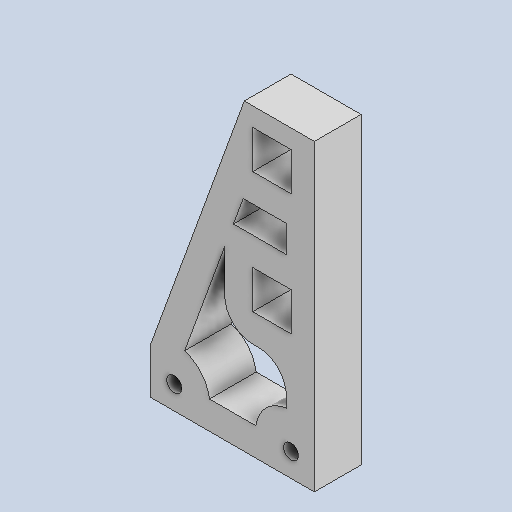
# Autodesk Inventor part: Soporte lateral
Saved by Autodesk Inventor 2024 (Build 280153000, 153)
## iProperties
Created: 2025-03-01
Part Number: Soporte lateral
Material: Genérico
Document SubType Name: Modeling
Designer: sergi
Density: 1 g/cm^3
Appearance: Valor por defecto
Author: sergi
Autodesk Inventor part; units mm, degrees
ref_plane "YZ Plane" through (0, 0, 0) normal (1, 0, 0) x (0, 1, 0)
ref_plane "XZ Plane" through (0, 0, 0) normal (0, 1, 0) x (-1, 0, 0)
ref_plane "XY Plane" through (0, 0, 0) normal (0, 0, 1) x (1, 0, 0)
sketch "Boceto1" plane through (0, 0, 0) normal (0, 0, 1) x (1, 0, 0)
  line L0 (0, 0) -> (105, 0)
  line L1 (105, 0) -> (105, 55)
  line L2 (105, 55) -> (0, 0)
  line L3 (105, 55) -> (90, 55)
  line L4 (90, 55) -> (0, 0)
  line L5 (0, 0) -> (70, 0)
  line L6 (70, 0) -> (90, 55)
  dimension "d0" = 105
  dimension "d1" = 55
  dimension "d4" = 15
  dimension "d10" = 70
  constraints: 14 end point, 2 horizontal, 1 perpendicular, 1 point on line
  measures "d0" distance of L0.start L0.end
  measures "d1" distance of L0.end L1.end
  measures "d4" distance of L1.end L3.end
  measures "d10" distance of L0.start L5.end
extrude "Extrusión1" add sketch "Boceto1" along normal blind 10 contours L6 L2 L1 L0 | L6 L3 L2
sketch "Boceto2" plane through (0, 0, 10) normal (0, 0, 1) x (1, 0, 0)
  line L0 (-10.0369, 16.82) -> (-5.1631, 16.82) projected
  line L1 (-1.5564, 16.82) -> (-5.1631, 16.82) projected
  line L2 (-1.5564, 16.82) -> (105, 16.82)
  line L3 (105, 0) -> (105, 55) projected
  line L4 (105, 55) -> (90, 55) projected
  line L5 (70, 0) -> (105, 0) projected
  line L6 (100, 5) -> (14.5727, 5)
  line L7 (90, 55) -> (70, 0) projected
  line L8 (105, 55) -> (105, 42.8)
  line L9 (105, 55) -> (117.2, 55) construction
  line L10 (70, 0) -> (105, 0) projected
  line L11 (105, 0) -> (105, 16.82)
  line L12 (105, 0) -> (105, 55) projected
  line L13 (105, 16.82) -> (100, 16.82)
  line L14 (100, 16.82) -> (94.1, 16.82)
  line L15 (94.1, 16.82) -> (94.1, 25.02)
  line L16 (94.1, 25.02) -> (100, 25.02)
  line L17 (100, 25.02) -> (100, 16.82)
  line L18 (105, 42.8) -> (100, 42.8)
  line L19 (100, 42.8) -> (91.8, 42.8)
  line L20 (91.8, 42.8) -> (91.8, 51)
  line L21 (91.8, 51) -> (100, 51)
  line L22 (100, 51) -> (100, 42.8)
  line L23 (100, 16.82) -> (91.8, 16.82)
  line L24 (91.8, 16.82) -> (91.8, 25.02)
  line L25 (91.8, 25.02) -> (100, 25.02)
  line L26 (100, 25.02) -> (100, 16.82)
  point P0 (0, 0)
  point P1 (94.1, 16.82)
  point P2 (100, 25.02)
  point P3 (91.8, 16.82)
  point P4 (105, 25.02)
  point P5 (162.8, 25.02)
  point P6 (162.8, 16.82)
  dimension "d22" = 90
  dimension "d25" = 8.2
  dimension "d26" = 12.2
  dimension "d27" = 8.2
  dimension "d28" = 8.2
  dimension "d31" = 8.2
  constraints: 38 end point, 6 horizontal, 6 parallel, 4 perpendicular, 3 collinear, 1 point on line
  measures "d22" angle of L8 L9
  measures "d25" distance of L14.end L15.end
  measures "d26" distance of L3.end L8.end
  measures "d27" distance of L20.end L21.end
  measures "d28" distance of L19.end L20.end
  measures "d31" distance of L24.end L25.end
extrude "Extrusión2" cut sketch "Boceto2" against normal through all contours L24 L25 L15 L2 | L15 L16 L17 L2 | L19 L20 L21 L22
sketch "Boceto3" plane through (70, 0, 0) normal (0, -1, 0) x (1, 0, 0)
  line L0 (21.8, 10) -> (21.8, 0) projected
  line L1 (0, 10) -> (35, 10) projected
  line L2 (0, 0) -> (35, 0) projected
  line L3 (35, 0) -> (35, 10) projected
  line L4 (0, 10) -> (0, 0) projected
  point P0 (-70, 0)
extrude "Extrusión3" add sketch "Boceto3" along normal blind 10
sketch "Boceto4" plane through (0, 0, 10) normal (0, 0, 1) x (1, 0, 0)
  circle A0 centre (100, -5) radius 2.1 projected
  circle A1 centre (75, -5) radius 2.1 projected
  point P0 (0, 0)
hole "Agujero1" at (75, -5, 10) at (100, -5, 10) direction (0, 0, -1) diameter 3.2 depth 10
shell "Vaciado1" thickness 6 removed faces 2 at (88.9333, 2.8793, 10) at (88.9333, 2.8793, 0)
fillet "Empalme1" radius 6 2 edges at (99, 10.82, 5) (85.8, 10.82, 5)
